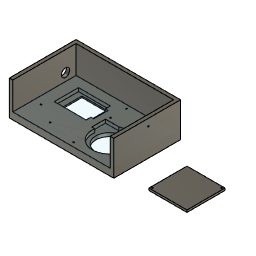
Case v5 (Autodesk Fusion 360 design; units mm, degrees)
Autodesk Fusion 360 part; units mm, degrees
sketch "Skizze1" plane through (0, 0, 0) normal (0, 0, 1) x (1, 0, 0)
  line L0 (0, 0) -> (141, 0)
  line L1 (141, 0) -> (141, 91.5)
  line L2 (141, 91.5) -> (0, 91.5)
  line L3 (0, 91.5) -> (0, 0)
  line L4 (25, 75) -> (61, 75)
  line L5 (61, 75) -> (61, 46)
  line L6 (61, 46) -> (25, 46)
  line L7 (25, 46) -> (25, 75)
  circle A0 centre (105, 35) radius 20
  dimension "d1" = 141
  dimension "d2" = 91.5
  dimension "d3" = 36
  dimension "d4" = 29
  dimension "d5" = 40
  constraint horizontal L0
  constraint vertical L1
  constraint horizontal L2
  constraint vertical L3
  constraint coincident L0.start L3.end
  constraint horizontal L4
  constraint vertical L5
  constraint horizontal L6
  constraint vertical L7
  measures "d1" distance of L0.start L0.end
  measures "d2" distance of L0.start L2.end
  measures "d3" distance of L4.start L4.end
  measures "d4" distance of L4.start L6.end
  measures "d5" diameter of A0
extrude "Extrusion1" add sketch "Skizze1" along normal blind 5 makes body 1
sketch "Skizze2" plane through (0, 0, 5) normal (0, 0, 1) x (-1, 0, 0)
  line L0 (-61, -46) -> (-25, -46)
  line L1 (-25, -46) -> (-25, -75)
  line L2 (-25, -75) -> (-61, -75)
  line L3 (-61, -75) -> (-61, -46)
  circle A0 centre (-105, -35) radius 20
  line L4 (0, -91.5) -> (0, 0)
  line L5 (0, 0) -> (-141, 0)
  line L6 (-141, 0) -> (-141, -91.5)
  line L7 (-141, -91.5) -> (0, -91.5)
  line L8 (-17, -78) -> (-67, -78)
  line L9 (-67, -78) -> (-67, -43)
  line L10 (-67, -43) -> (-17, -43)
  line L11 (-17, -43) -> (-17, -78)
  circle A1 centre (-105, -35) radius 25
  dimension "d8" = 50
  dimension "d9" = 35
  dimension "d10" = 6
  dimension "d11" = 50
  constraint horizontal L8
  constraint vertical L9
  constraint horizontal L10
  constraint vertical L11
  constraint concentric A0 A1
  measures "d8" distance of L8.start L8.end
  measures "d9" distance of L8.start L10.end
  measures "d10" horizontal distance of L2.end L8.end
  measures "d11" diameter of A1
extrude "Extrusion2" add sketch "Skizze2" along normal blind 5 contours L4 L5 L6 L7 bodies 1
sketch "Skizze3" plane through (0, 0, 5) normal (0, 0, 1) x (-1, 0, 0)
  line L0 (-61, -46) -> (-25, -46)
  line L1 (-25, -46) -> (-25, -75)
  line L2 (-25, -75) -> (-61, -75)
  line L3 (-61, -75) -> (-61, -46)
  line L4 (-67, -43) -> (-67, -78)
  line L5 (-67, -78) -> (-17, -78)
  line L6 (-17, -78) -> (-17, -43)
  line L7 (-17, -43) -> (-67, -43)
  line L8 (-61, -78) -> (-67, -78)
  line L9 (-67, -78) -> (-67, -71)
  line L10 (-67, -71) -> (-61, -71)
  line L11 (-61, -71) -> (-61, -78)
  line L12 (-67, -43) -> (-61, -43)
  line L13 (-61, -43) -> (-61, -50)
  line L14 (-61, -50) -> (-67, -50)
  line L15 (-67, -50) -> (-67, -43)
  dimension "d14" = 6
  dimension "d15" = 7
  dimension "d16" = 7
  dimension "d17" = 21
  constraint horizontal L8
  constraint vertical L9
  constraint horizontal L10
  constraint vertical L11
  constraint coincident L4 L9.end
  constraint coincident L5 L8.start
  constraint horizontal L12
  constraint vertical L13
  constraint horizontal L14
  constraint vertical L15
  constraint coincident L3 L13.end
  constraint coincident L4.start L7.end
  measures "d14" distance of L8.start L4.end
  measures "d15" distance of L8.start L10.end
  measures "d16" distance of L12.end L13.end
  measures "d17" distance of L10.end L13.end
extrude "Extrusion3" add sketch "Skizze3" along normal blind 5 contours L3 L4 L7 L12 L13 L14 L15 | L3 L4 L5 L8 L9 L10 L11 bodies 1
sketch "Skizze4" plane through (0, 0, 10) normal (0, 0, 1) x (-1, 0, 0)
  line L0 (-61, -43) -> (-17, -43)
  line L1 (-17, -43) -> (-17, -78)
  line L2 (-17, -78) -> (-61, -78)
  line L3 (-61, -78) -> (-61, -71)
  line L4 (-61, -71) -> (-67, -71)
  line L5 (-67, -71) -> (-67, -50)
  line L6 (-67, -50) -> (-61, -50)
  line L7 (-61, -50) -> (-61, -43)
  circle A0 centre (-105, -35) radius 25
  line L8 (-141, -91.5) -> (0, -91.5)
  line L9 (0, -91.5) -> (0, 0)
  line L10 (0, 0) -> (-141, 0)
  line L11 (-141, 0) -> (-141, -91.5)
extrude "Extrusion4" add 1 faces at (141, 30.5, 3.3333) along direction (1, 0, 0) blind 5 on bodies 1 bodies 1
extrude "Extrusion5" add 1 faces at (0, 61, 3.3333) along direction (-1, 0, 0) blind 5 on bodies 1 bodies 1
extrude "Extrusion6" add 1 faces at (95.6667, 91.5, 6.6667) along direction (0, 1, 0) blind 5 on bodies 1 bodies 1
sketch "Skizze5" plane through (0, 0, 10) normal (0, 0, 1) x (-1, 0, 0)
  line L0 (-61, -43) -> (-17, -43)
  line L1 (-17, -43) -> (-17, -78)
  line L2 (-17, -78) -> (-61, -78)
  line L3 (-61, -78) -> (-61, -71)
  line L4 (-61, -71) -> (-67, -71)
  line L5 (-67, -71) -> (-67, -50)
  line L6 (-67, -50) -> (-61, -50)
  line L7 (-61, -50) -> (-61, -43)
  circle A0 centre (-105, -35) radius 25
  line L8 (5, -96.5) -> (5, 0)
  line L9 (5, 0) -> (-146, 0)
  line L10 (-146, 0) -> (-146, -96.5)
  line L11 (-146, -96.5) -> (5, -96.5)
  line L12 (0, 0) -> (-141, 0)
  line L13 (-141, 0) -> (-141, -91.5)
  line L14 (-141, -91.5) -> (0, -91.5)
  line L15 (0, -91.5) -> (0, 0)
  point P0 (0, -91.5)
  dimension "d27" = 5
  dimension "d28" = 5
  dimension "d29" = 141
  constraint horizontal L12
  constraint vertical L13
  constraint horizontal L14
  constraint vertical L15
  constraint coincident L12.start L15.end
  measures "d27" vertical distance of L8.start P0
  measures "d28" distance of L8 P0
  measures "d29" distance of L13.end P0
extrude "Extrusion7" add sketch "Skizze5" along normal blind 30 contours L8 L9 L10 L11 L13 L14 L15 bodies 1
sketch "Skizze6" plane through (146, 0, 0) normal (1, 0, 0) x (0, 1, 0)
  line L0 (0, 0) -> (96.5, 0)
  line L1 (96.5, 0) -> (96.5, 40)
  line L2 (96.5, 40) -> (0, 40)
  line L3 (0, 40) -> (0, 0)
  circle A0 centre (50, 26) radius 1
  dimension "d32" = 2
  dimension "d33" = 14
  measures "d32" diameter of A0
  measures "d33" distance of L2 A0.centre
hole "Bohrung1" at (146, 50, 26) direction (-1, 0, 0) diameter 2 depth 15 tip angle 118 bodies 1
sketch "Skizze7" plane through (0, 0, 10) normal (0, 0, 1) x (1, 0, 0)
  circle A0 centre (136, 86.5) radius 1
  line L0 (141, 91.5) -> (0, 91.5)
  line L1 (141, 0) -> (141, 91.5)
  circle A1 centre (136, 63.5) radius 1
  circle A2 centre (78, 63.5) radius 1
  circle A3 centre (78, 86.5) radius 1
  dimension "d37" = 2
  dimension "d38" = 5
  dimension "d39" = 5
  dimension "d40" = 2
  dimension "d41" = 23
  dimension "d42" = 5
  dimension "d43" = 2
  dimension "d44" = 58
  dimension "d45" = 2
  constraint vertical A0.centre A1.centre
  constraint horizontal A1.centre A2.centre
  constraint vertical A2.centre A3.centre
  constraint horizontal A0.centre A3.centre
  measures "d37" diameter of A0
  measures "d38" distance of A0.centre L0
  measures "d39" distance of A0.centre L1
  measures "d40" diameter of A1
  measures "d41" distance of A0.centre A1.centre
  measures "d42" distance of L1 A1.centre
  measures "d43" diameter of A2
  measures "d44" horizontal distance of A1.centre A2.centre
  measures "d45" diameter of A3
extrude "Extrusion8" cut sketch "Skizze7" against normal blind 7 bodies 1
sketch "Skizze8" plane through (0, 0, 10) normal (0, 0, 1) x (-1, 0, 0)
  line L0 (-76, -58) -> (-95.5417, -58)
  line L1 (-95.5417, -58) -> (-95.5417, -38.3516)
  line L2 (-95.5417, -38.3516) -> (-76, -38.3516)
  line L3 (-76, -38.3516) -> (-76, -58)
  constraint horizontal L0
  constraint vertical L1
  constraint horizontal L2
  constraint vertical L3
extrude "Extrusion9" cut sketch "Skizze8" against normal blind 5 bodies 1
sketch "Skizze9" plane through (0, 0, 0) normal (1, 0, 0) x (0, 1, 0)
sketch "Skizze10" plane through (0, 0, 0) normal (0, 0, 1) x (1, 0, 0)
  line L0 (175, 75) -> (235, 75)
  line L1 (235, 75) -> (235, 15)
  line L2 (235, 15) -> (175, 15)
  line L3 (175, 15) -> (175, 75)
  circle A0 centre (230, 70) radius 1
  circle A1 centre (180, 20) radius 1
  dimension "d50" = 60
  dimension "d51" = 60
  dimension "d52" = 2
  dimension "d53" = 2
  constraint horizontal L0
  constraint vertical L1
  constraint horizontal L2
  constraint vertical L3
  measures "d50" distance of L0.start L0.end
  measures "d51" distance of L0.start L2.end
  measures "d52" diameter of A0
  measures "d53" diameter of A1
sketch "Skizze11" plane through (0, 0, 10) normal (0, 0, 1) x (1, 0, 0)
  circle A0 centre (132, 58) radius 1
  circle A1 centre (82, 8) radius 1
  line L0 (186.7679, 65.1213) -> (241.7679, 65.1213)
  line L1 (241.7679, 65.1213) -> (241.7679, 10.1213)
  line L2 (241.7679, 10.1213) -> (186.7679, 10.1213)
  line L3 (186.7679, 10.1213) -> (186.7679, 65.1213)
  circle A2 centre (239, 63) radius 1
  circle A3 centre (189, 13) radius 1
  dimension "d56" = 2
  dimension "d57" = 2
  dimension "d58" = 50
  dimension "d59" = 50
  dimension "d60" = 55
  dimension "d61" = 55
  dimension "d62" = 2
  dimension "d63" = 2
  dimension "d64" = 50
  dimension "d65" = 50
  constraint horizontal L0
  constraint vertical L1
  constraint horizontal L2
  constraint vertical L3
  measures "d56" diameter of A0
  measures "d57" diameter of A1
  measures "d58" vertical distance of A0.centre A1.centre
  measures "d59" horizontal distance of A0.centre A1.centre
  measures "d60" distance of L0.start L0.end
  measures "d61" distance of L0.start L2.end
  measures "d62" diameter of A2
  measures "d63" diameter of A3
  measures "d64" horizontal distance of A2.centre A3.centre
  measures "d65" vertical distance of A2.centre A3.centre
extrude "Extrusion11" add sketch "Skizze11" along normal blind 3 separate body contours L0 L1 L2 L3 makes body 2
move_body "Verschieben1" bodies 2 to x (1, 0, 0) y (0, 1, 0) z (0, 0, 1) at (0, 0, -10)
sketch "Skizze12" plane through (61, 0, 0) normal (-1, 0, 0) x (0, -1, 0)
  line L0 (-75, 0) -> (-46, 0)
  line L1 (-46, 0) -> (-46, 5)
  line L2 (-46, 5) -> (-43, 5)
  line L3 (-43, 5) -> (-43, 10)
  line L4 (-43, 10) -> (-50, 10)
  line L5 (-50, 10) -> (-50, 5)
  line L6 (-50, 5) -> (-71, 5)
  line L7 (-71, 5) -> (-71, 10)
  line L8 (-71, 10) -> (-78, 10)
  line L9 (-78, 10) -> (-78, 5)
  line L10 (-78, 5) -> (-75, 5)
  line L11 (-75, 5) -> (-75, 0)
  line L12 (-50, 10) -> (-43, 10)
  line L13 (-43, 10) -> (-43, 5)
  line L14 (-43, 5) -> (-50, 5)
  line L15 (-50, 5) -> (-50, 10)
  line L16 (-71, 10) -> (-78, 10)
  line L17 (-78, 10) -> (-78, 5)
  line L18 (-78, 5) -> (-71, 5)
  line L19 (-71, 5) -> (-71, 10)
  constraint horizontal L12
  constraint vertical L13
  constraint horizontal L14
  constraint vertical L15
  constraint coincident L2.end L3.start
  constraint coincident L4.end L5.start
  constraint horizontal L16
  constraint vertical L17
  constraint horizontal L18
  constraint vertical L19
  constraint coincident L9.end L10.start
  constraint coincident L7.end L8.start
extrude "Extrusion12" cut sketch "Skizze12" against normal blind 2 contours L7 L8 L9 L10 L16 L17 L18 L19 | L2 L3 L4 L5 L12 L13 L14 L15 bodies 1
sketch "Skizze13" plane through (0, 0, 10) normal (0, 0, 1) x (1, 0, 0)
  circle A0 centre (11, 30) radius 1
  circle A1 centre (40, 14) radius 1
  dimension "d70" = 2
  dimension "d71" = 2
  dimension "d72" = 29
  dimension "d73" = 16
  measures "d70" diameter of A0
  measures "d71" diameter of A1
  measures "d72" horizontal distance of A0.centre A1.centre
  measures "d73" vertical distance of A0.centre A1.centre
extrude "Extrusion13" cut sketch "Skizze13" against normal blind 7 bodies 1
extrude "Extrusion14" add 1 faces at (94, 94.8333, 40) along direction (0, 0, 1) blind 10 on bodies 1 bodies 1
sketch "Skizze14" plane through (146, 0, 0) normal (1, 0, 0) x (0, 1, 0)
  circle A0 centre (50, 26) radius 1
  line L0 (0, 0) -> (96.5, 0)
  line L1 (96.5, 0) -> (96.5, 50)
  line L2 (96.5, 50) -> (0, 50)
  line L3 (0, 50) -> (0, 0)
  circle A1 centre (50, 40) radius 1
  dimension "d78" = 2
  dimension "d79" = 10
  measures "d78" diameter of A1
  measures "d79" distance of L2 A1.centre
extrude "Extrusion15" cut sketch "Skizze14" against normal blind 20 contours A1 bodies 1
sketch "Skizze15" plane through (146, 0, 0) normal (1, 0, 0) x (0, 1, 0)
  circle A0 centre (50, 40) radius 1
  circle A1 centre (50, 26) radius 1
  line L0 (0, 0) -> (96.5, 0)
  line L1 (96.5, 0) -> (96.5, 50)
  line L2 (96.5, 50) -> (0, 50)
  line L3 (0, 50) -> (0, 0)
extrude "Extrusion16" add sketch "Skizze15" against normal blind 5 contours A1 bodies 1
sketch "Skizze16" plane through (0, 0, 10) normal (0, 0, 1) x (1, 0, 0)
  circle A0 centre (132, 56) radius 1
  circle A1 centre (82, 6) radius 1
  dimension "d84" = 2
  dimension "d85" = 2
  dimension "d86" = 50
  dimension "d87" = 50
  measures "d84" diameter of A0
  measures "d85" diameter of A1
  measures "d86" horizontal distance of A0.centre A1.centre
  measures "d87" vertical distance of A0.centre A1.centre
extrude "Extrusion17" cut sketch "Skizze16" against normal blind 7 bodies 1
sketch "Skizze17" plane through (0, 0, 0) normal (0, 0, -1) x (1, 0, 0)
  line L0 (25, -46) -> (61, -46)
  line L1 (61, -46) -> (61, -75)
  line L2 (61, -75) -> (25, -75)
  line L3 (25, -75) -> (25, -46)
  circle A0 centre (105, -35) radius 20
  line L4 (146, -96.5) -> (146, 0)
  line L5 (146, 0) -> (-5, 0)
  line L6 (-5, 0) -> (-5, -96.5)
  line L7 (-5, -96.5) -> (146, -96.5)
  line L8 (15, -36) -> (71, -36)
  line L9 (71, -36) -> (71, -85)
  line L10 (71, -85) -> (15, -85)
  line L11 (15, -85) -> (15, -36)
  dimension "d90" = 10
  dimension "d91" = 10
  dimension "d92" = 10
  dimension "d93" = 10
  constraint horizontal L8
  constraint vertical L9
  constraint horizontal L10
  constraint vertical L11
  measures "d90" distance of L0.start L11
  measures "d91" distance of L0.start L8
  measures "d92" distance of L2.end L10
  measures "d93" distance of L0.end L9
extrude "Extrusion18" cut sketch "Skizze17" against normal blind 3 contours L8 L9 L10 L11 bodies 1
sketch "Skizze18" plane through (0, 0, 10) normal (0, 0, 1) x (-1, 0, 0)
hole "Bohrung2" at (0, 76.3167, 21.0886) direction (-1, 0, 0) diameter 12 depth 30 tip angle 118 bodies 1
